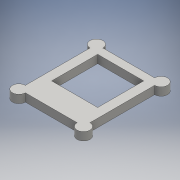
# Autodesk Inventor part: cubierta OLED
Saved by Autodesk Inventor 2016 (Build 200138000, 138)
## iProperties
Created: 2017-05-09
Part Number: cubierta OLED
Material: Generic
Document SubType Name: Modeling
Designer: rdiaz
Density: 1 g/cm^3
Appearance: Default
Author: rdiaz
Autodesk Inventor part; units mm, degrees
ref_plane "YZ Plane" through (0, 0, 0) normal (1, 0, 0) x (0, 1, 0)
ref_plane "XZ Plane" through (0, 0, 0) normal (0, 1, 0) x (-1, 0, 0)
ref_plane "XY Plane" through (0, 0, 0) normal (0, 0, 1) x (1, 0, 0)
sketch "Sketch1" plane through (0, 0, 0) normal (0, 0, 1) x (1, 0, 0)
  line L0 (-20, 24) -> (20, 24)
  line L1 (20, 24) -> (20, -24)
  line L2 (20, -24) -> (-20, -24)
  line L3 (-20, -24) -> (-20, 24)
  line L4 (-14.25, 19) -> (14.25, 19)
  line L5 (14.25, 19) -> (14.25, -9.5)
  line L6 (14.25, -9.5) -> (-14.25, -9.5)
  line L7 (-14.25, -9.5) -> (-14.25, 19)
  circle A0 centre (-20, 24) radius 4
  circle A1 centre (20, 24) radius 4
  circle A2 centre (20, -24) radius 4
  circle A3 centre (-20, -24) radius 4
  point P0 (20, 0)
  point P1 (0, 24)
  point P2 (0, 0)
  point P3 (-20, 0)
  point P4 (0, 19)
  dimension "d0" = 40
  dimension "d1" = 48
  dimension "d3" = 5
  dimension "d4" = 28.5
  dimension "d5" = 28.5
  dimension "d8" = 8
  dimension "d9" = 8
  dimension "d10" = 8
  dimension "d11" = 8
  constraints: 16 end point, 4 centre point, 4 coincident, 4 midpoint, 4 parallel, 2 horizontal, 2 perpendicular, 2 vertical alignment, 1 horizontal alignment
  measures "d0" distance of L0.start L0.end
  measures "d1" distance of L0.end L1.end
  measures "d3" distance between parallel lines of L4 L0
  measures "d4" distance of L4.start L4.end
  measures "d5" distance of L6.end L4.start
  measures "d8" diameter of A0
  measures "d9" diameter of A1
  measures "d10" diameter of A2
  measures "d11" diameter of A3
extrude "Extrusion1" add sketch "Sketch1" along normal blind 5
body "Solid1"
